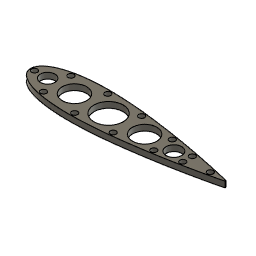
rib_spar (Autodesk Fusion 360 design; units mm, degrees)
Autodesk Fusion 360 part; units mm, degrees
sketch "Sketch1" plane through (0, 0, 0) normal (0, 1, 0) x (1, 0, 0)
  circle A0 centre (45, 0) radius 12.5
  circle A1 centre (147, 0) radius 8
  circle A2 centre (117, 0) radius 12.5
  circle A3 centre (17.5, 0) radius 7.5
  spline S0 degree 5 poles (200, 0.442) (199.5349, 0.5546) (198.6142, 0.7771) (197.2617, 1.103) (195.5156, 1.5218) (193.4243, 2.0198) (191.4115, 2.495) (189.4526, 2.9528) (187.5051, 3.4019) (185.509, 3.8552) (183.3993, 4.3263) (181.1175, 4.8274) (178.6226, 5.3668) (175.9043, 5.946) (172.9837, 6.5597) (169.9021, 7.1983) (166.7141, 7.8492) (163.4783, 8.4993) (160.249, 9.1365) (157.0682, 9.7517) (153.9563, 10.3407) (150.9161, 10.9035) (147.9371, 11.4428) (145.0001, 11.9633) (142.0821, 12.4703) (139.1599, 12.9686) (136.2156, 13.4615) (133.2392, 13.95) (130.2271, 14.4333) (127.1814, 14.9094) (124.1082, 15.3759) (121.0171, 15.83) (117.9195, 16.2692) (114.8283, 16.6922) (111.7556, 17.0983) (108.7119, 17.4875) (105.7037, 17.8601) (102.7328, 18.2165) (99.7938, 18.557) (96.8732, 18.8812) (93.9476, 19.1882) (90.9896, 19.4767) (87.9733, 19.7449) (84.8792, 19.9909) (81.7005, 20.213) (78.4473, 20.4095) (75.154, 20.5792) (71.8773, 20.7215) (68.6831, 20.836) (65.6373, 20.9226) (62.7944, 20.9816) (60.1868, 21.0131) (57.815, 21.0176) (55.6351, 20.9954) (53.5753, 20.9468) (51.5571, 20.8725) (49.5124, 20.7736) (47.4055, 20.652) (45.2448, 20.5097) (43.061, 20.3486) (40.8911, 20.1683) (38.7615, 19.966) (36.6665, 19.7341) (34.5722, 19.4623) (32.439, 19.1408) (30.239, 18.7629) (27.9748, 18.3286) (25.7002, 17.8477) (23.4982, 17.3363) (21.4536, 16.8128) (19.6289, 16.2935) (18.0357, 15.7888) (16.6175, 15.2995) (15.2858, 14.8132) (13.9485, 14.303) (12.5439, 13.7217) (11.0505, 13.0221) (9.4884, 12.1818) (7.9289, 11.2337) (6.4838, 10.2684) (5.2468, 9.368) (4.2539, 8.5628) (3.414, 7.7584) (2.5815, 6.7898) (1.6751, 5.516) (0.7924, 3.9084) (0.1283, 2.0295) (-0.1251, 0) (0.1283, -2.0295) (0.7924, -3.9084) (1.6751, -5.516) (2.5815, -6.7898) (3.414, -7.7584) (4.2539, -8.5628) (5.2468, -9.368) (6.4838, -10.2684) (7.9289, -11.2337) (9.4884, -12.1818) (11.0505, -13.0221) (12.5439, -13.7217) (13.9485, -14.303) (15.2858, -14.8132) (16.6175, -15.2995) (18.0357, -15.7888) (19.6289, -16.2935) (21.4536, -16.8128) (23.4982, -17.3363) (25.7002, -17.8477) (27.9748, -18.3286) (30.239, -18.7629) (32.439, -19.1408) (34.5722, -19.4623) (36.6665, -19.7341) (38.7615, -19.966) (40.8911, -20.1683) (43.061, -20.3486) (45.2448, -20.5097) (47.4055, -20.652) (49.5124, -20.7736) (51.5571, -20.8725) (53.5753, -20.9468) (55.6351, -20.9954) (57.815, -21.0176) (60.1868, -21.0131) (62.7944, -20.9816) (65.6373, -20.9226) (68.6831, -20.836) (71.8773, -20.7215) (75.154, -20.5792) (78.4473, -20.4095) (81.7005, -20.213) (84.8792, -19.9909) (87.9733, -19.7449) (90.9896, -19.4767) (93.9476, -19.1882) (96.8732, -18.8812) (99.7938, -18.557) (102.7328, -18.2165) (105.7037, -17.8601) (108.7119, -17.4875) (111.7556, -17.0983) (114.8283, -16.6922) (117.9195, -16.2692) (121.0171, -15.83) (124.1082, -15.3759) (127.1814, -14.9094) (130.2271, -14.4333) (133.2392, -13.95) (136.2156, -13.4615) (139.1599, -12.9686) (142.0821, -12.4703) (145.0001, -11.9633) (147.9371, -11.4428) (150.9161, -10.9035) (153.9563, -10.3407) (157.0682, -9.7517) (160.249, -9.1365) (163.4783, -8.4993) (166.7141, -7.8492) (169.9021, -7.1983) (172.9837, -6.5597) (175.9043, -5.946) (178.6226, -5.3668) (181.1175, -4.8274) (183.3993, -4.3263) (185.509, -3.8552) (187.5051, -3.4019) (189.4526, -2.9528) (191.4115, -2.495) (193.4243, -2.0198) (195.5156, -1.5218) (197.2617, -1.103) (198.6142, -0.7771) (199.5349, -0.5546) (200, -0.442) knots 0 0 0 0 0 0 0.00588235 0.01176471 0.01764706 0.02352941 0.02941176 0.03529412 0.04117647 0.04705882 0.05294118 0.05882353 0.06470588 0.07058824 0.07647059 0.08235294 0.08823529 0.09411765 0.1 0.10588235 0.11176471 0.11764706 0.12352941 0.12941176 0.13529412 0.14117647 0.14705882 0.15294118 0.15882353 0.16470588 0.17058824 0.17647059 0.18235294 0.18823529 0.19411765 0.2 0.20588235 0.21176471 0.21764706 0.22352941 0.22941176 0.23529412 0.24117647 0.24705882 0.25294118 0.25882353 0.26470588 0.27058824 0.27647059 0.28235294 0.28823529 0.29411765 0.3 0.30588235 0.31176471 0.31764706 0.32352941 0.32941176 0.33529412 0.34117647 0.34705882 0.35294118 0.35882353 0.36470588 0.37058824 0.37647059 0.38235294 0.38823529 0.39411765 0.4 0.40588235 0.41176471 0.41764706 0.42352941 0.42941176 0.43529412 0.44117647 0.44705882 0.45294118 0.45882353 0.46470588 0.47058824 0.47647059 0.48235294 0.48823529 0.49411765 0.5 0.50588235 0.51176471 0.51764706 0.52352941 0.52941176 0.53529412 0.54117647 0.54705882 0.55294118 0.55882353 0.56470588 0.57058824 0.57647059 0.58235294 0.58823529 0.59411765 0.6 0.60588235 0.61176471 0.61764706 0.62352941 0.62941176 0.63529412 0.64117647 0.64705882 0.65294118 0.65882353 0.66470588 0.67058824 0.67647059 0.68235294 0.68823529 0.69411765 0.7 0.70588235 0.71176471 0.71764706 0.72352941 0.72941176 0.73529412 0.74117647 0.74705882 0.75294118 0.75882353 0.76470588 0.77058824 0.77647059 0.78235294 0.78823529 0.79411765 0.8 0.80588235 0.81176471 0.81764706 0.82352941 0.82941176 0.83529412 0.84117647 0.84705882 0.85294118 0.85882353 0.86470588 0.87058824 0.87647059 0.88235294 0.88823529 0.89411765 0.9 0.90588235 0.91176471 0.91764706 0.92352941 0.92941176 0.93529412 0.94117647 0.94705882 0.95294118 0.95882353 0.96470588 0.97058824 0.97647059 0.98235294 0.98823529 0.99411765 1 1 1 1 1 1
  line L0 (0, 0) -> (200, 0) construction
  line L1 (200, 0.442) -> (200, -0.442)
  circle A4 centre (80, 0) radius 15
  spline S1 degree 3 poles (184.4124, 0) (182.9803, 0.3219) (181.4614, 0.6576) (179.7797, 1.0229) (176.9402, 1.6396) (173.6059, 2.3469) (169.9798, 3.0958) (165.9314, 3.9319) (161.5916, 4.8034) (157.4548, 5.6011) (152.8951, 6.4803) (148.584, 7.2703) (144.3663, 8.0109) (139.7657, 8.8186) (135.1906, 9.5885) (130.4523, 10.3442) (123.6067, 11.436) (116.4669, 12.4627) (109.5737, 13.3431) (104.9199, 13.9376) (100.4212, 14.4752) (95.9565, 14.9522) (91.9415, 15.3811) (87.8921, 15.7592) (83.5692, 16.0684) (79.6892, 16.346) (75.5661, 16.5669) (71.5968, 16.7233) (67.9067, 16.8687) (64.4155, 16.9587) (61.4503, 16.9945) (58.5497, 17.0294) (56.1674, 17.0128) (53.9118, 16.9482) (51.8555, 16.8893) (49.8299, 16.7896) (47.6689, 16.6563) (44.9728, 16.49) (42.1555, 16.2794) (39.5095, 16.0132) (37.1245, 15.7733) (34.8436, 15.4796) (32.4025, 15.0696) (30.0744, 14.6785) (27.5585, 14.1731) (25.2539, 13.6312) (23.3903, 13.1929) (21.7256, 12.7425) (20.3526, 12.3191) (18.7468, 11.8238) (17.4519, 11.3571) (16.1277, 10.8492) (14.8261, 10.3499) (13.5355, 9.8063) (12.1365, 9.051) (10.7812, 8.3192) (9.3198, 7.3742) (8.2433, 6.5911) (7.5659, 6.0984) (7.0731, 5.6983) (6.692, 5.3392) (6.3313, 4.9993) (6.012, 4.6492) (5.6343, 4.1426) (5.0278, 3.3292) (4.3695, 2.1551) (4.1257, 1.0839) (3.9158, 0.1615) (3.9673, -0.6872) (4.278, -1.6286) (4.6332, -2.7048) (5.3337, -3.7884) (5.905, -4.4903) (6.4182, -5.1209) (6.8092, -5.488) (7.5542, -6.0721) (8.5083, -6.8201) (10.0326, -7.8602) (11.5167, -8.7068) (12.8911, -9.4909) (14.1824, -10.0782) (15.444, -10.5819) (16.7338, -11.0968) (17.9879, -11.5547) (19.4428, -12.0301) (20.6562, -12.4267) (22.0761, -12.8418) (23.7463, -13.2638) (26.0244, -13.8395) (28.6859, -14.4087) (31.1756, -14.8562) (34.1738, -15.3951) (36.9113, -15.7575) (39.7972, -16.0418) (42.3436, -16.2927) (45.0447, -16.494) (47.6321, -16.654) (49.7178, -16.783) (51.6812, -16.8808) (53.6597, -16.9408) (55.8183, -17.0062) (58.0673, -17.0276) (60.7821, -17.0017) (63.7053, -16.9738) (67.1704, -16.8908) (70.8758, -16.7511) (74.7017, -16.6069) (78.7138, -16.4019) (82.5104, -16.1425) (87.2145, -15.8211) (91.5961, -15.4177) (95.928, -14.9552) (100.3718, -14.4808) (104.848, -13.9461) (109.4784, -13.3553) (116.4467, -12.4661) (123.6691, -11.4272) (130.5882, -10.3225) (135.3603, -9.5605) (139.9654, -8.7849) (144.6034, -7.9692) (148.506, -7.2828) (152.4881, -6.5542) (156.6842, -5.7493) (161.1472, -4.8932) (165.872, -3.9453) (170.2461, -3.0408) (173.7241, -2.3216) (176.9247, -1.6425) (179.6686, -1.047) (181.3943, -0.6724) (182.9494, -0.3288) (184.4124, 0) knots 0.04172113 0.04172113 0.04172113 0.04172113 0.05400533 0.05400533 0.05400533 0.07474533 0.07474533 0.07474533 0.09790022 0.09790022 0.09790022 0.1234227 0.1234227 0.1234227 0.15126136 0.15126136 0.15126136 0.19148069 0.19148069 0.19148069 0.21863333 0.21863333 0.21863333 0.24305103 0.24305103 0.24305103 0.26496763 0.26496763 0.26496763 0.28534254 0.28534254 0.28534254 0.30527482 0.30527482 0.30527482 0.32344559 0.32344559 0.32344559 0.34611618 0.34611618 0.34611618 0.36655005 0.36655005 0.36655005 0.38603819 0.38603819 0.38603819 0.40179701 0.40179701 0.40179701 0.42022827 0.42022827 0.42022827 0.43834614 0.43834614 0.43834614 0.45589782 0.45589782 0.45589782 0.46694207 0.46694207 0.46694207 0.47739535 0.47739535 0.47739535 0.49417982 0.49417982 0.49417982 0.50863257 0.50863257 0.50863257 0.52515315 0.52515315 0.52515315 0.53999212 0.53999212 0.53999212 0.55899528 0.55899528 0.55899528 0.57659435 0.57659435 0.57659435 0.59458653 0.59458653 0.59458653 0.60959153 0.60959153 0.60959153 0.63005789 0.63005789 0.63005789 0.65470418 0.65470418 0.65470418 0.67645125 0.67645125 0.67645125 0.69398167 0.69398167 0.69398167 0.71310782 0.71310782 0.71310782 0.73370127 0.73370127 0.73370127 0.7549639 0.7549639 0.7549639 0.781309 0.781309 0.781309 0.80833393 0.80833393 0.80833393 0.84900501 0.84900501 0.84900501 0.87705558 0.87705558 0.87705558 0.90065833 0.90065833 0.90065833 0.92576342 0.92576342 0.92576342 0.94572484 0.94572484 0.94572484 0.95827887 0.95827887 0.95827887 0.95827887
  circle A5 centre (27.3331, -14.0977) radius 3
  circle A6 centre (3.9991, 0) radius 3
  circle A7 centre (62.2515, -16.9837) radius 3
  circle A8 centre (99.338, -14.5803) radius 3
  circle A9 centre (135.9448, -9.4502) radius 3
  circle A10 centre (161.0623, -4.8971) radius 3
  circle A11 centre (184.4124, 0) radius 3
  circle A12 centre (27.3331, 14.0977) radius 3
  circle A13 centre (62.2515, 16.9837) radius 3
  circle A14 centre (99.338, 14.5803) radius 3
  circle A15 centre (135.9448, 9.4502) radius 3
  circle A16 centre (161.0623, 4.8971) radius 3
  point P0 (160, -9.182)
  point P1 (140, -12.824)
  point P2 (190, -2.824)
  point P3 (180, -5.068)
  point P4 (15, 14.7)
  point P5 (10, -12.442)
  point P6 (2.5, 6.63)
  point P7 (5, 9.152)
  point P8 (10, 12.442)
  point P9 (100, -18.53)
  point P10 (5, -9.152)
  point P11 (2.5, -6.63)
  point P12 (50, 20.794)
  point P13 (30, 18.708)
  point P14 (20, 16.39)
  point P15 (40, 20.08)
  point P16 (60, -21.008)
  point P17 (80, -20.312)
  point P18 (180, 5.068)
  point P19 (190, 2.824)
  point P20 (20, -16.39)
  point P21 (30, -18.708)
  point P22 (40, -20.08)
  point P23 (50, -20.794)
  point P24 (120, 15.972)
  point P25 (100, 18.53)
  point P26 (80, 20.312)
  point P27 (60, 21.008)
  point P28 (140, 12.824)
  point P29 (160, 9.182)
  point P30 (15, -14.7)
  point P31 (120, -15.972)
  point P32 (161.0623, 4.8971)
  dimension "d14" = 25
  dimension "d15" = 16
  dimension "d16" = 25
  dimension "d17" = 30
  dimension "d30" = -4
  dimension "d31" = 6
  dimension "d32" = 6
  dimension "d33" = 6
  dimension "d34" = 6
  dimension "d35" = 6
  dimension "d36" = 6
  dimension "d37" = 6
  constraint coincident L0.start origin
  constraint horizontal L0
  constraint perpendicular L0 L1
  constraint coincident A0.centre L0
  constraint coincident A1.centre L0
  constraint coincident A2.centre L0
  constraint coincident A4.centre L0
  constraint coincident S1 A5.centre
  constraint coincident S1 A7.centre
  constraint coincident S1 A8.centre
  constraint coincident S1 A9.centre
  constraint coincident S1 A6.centre
  constraint coincident L0 A6.centre
  constraint coincident S1 A10.centre
  constraint coincident S1 A11.centre
  constraint symmetric L0 A5 A12
  constraint symmetric L0 A7 A13
  constraint symmetric L0 A8 A14
  constraint symmetric L0 A9 A15
  constraint symmetric L0 A10.centre P32
  constraint symmetric L0 A10 A16
  measures "d14" diameter of A0
  measures "d15" diameter of A1
  measures "d16" diameter of A2
  measures "d17" diameter of A4
  measures "d31" diameter of A5
  measures "d32" diameter of A6
  measures "d33" diameter of A7
  measures "d34" diameter of A8
  measures "d35" diameter of A9
  measures "d36" diameter of A10
  measures "d37" diameter of A11
extrude "Extrude2" add sketch "Sketch1" along normal blind 6 contours A1 S1 A10 A11 A16 | A1 A2 S1 A9 A15 | A2 S1 A5 A6 A7 A8 A12 A13 A14 | S0 L1
